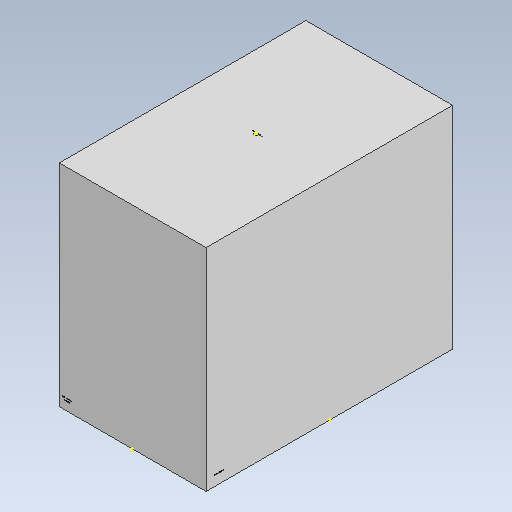
# Autodesk Inventor part: wheelchair_extended_box
Saved by Autodesk Inventor 2021 (Build 250183000, 183)
## iProperties
Created: 2021-05-27
Part Number: wheelchair_extended_box
Material: Generic
Document SubType Name: Modeling
Designer: Watchdog
Density: 1 g/cm^3
Appearance: Default
Author: Watchdog
Autodesk Inventor part; units mm, degrees
ref_plane "YZ Plane" through (0, 0, 0) normal (1, 0, 0) x (0, 1, 0)
ref_plane "XZ Plane" through (0, 0, 0) normal (0, 1, 0) x (-1, 0, 0)
ref_plane "XY Plane" through (0, 0, 0) normal (0, 0, 1) x (1, 0, 0)
sketch "Sketch1" plane through (0, 0, 0) normal (0, 1, 0) x (-1, 0, 0)
  line L0 (317.5, -533.5) -> (-317.5, -533.5)
  line L1 (-317.5, -533.5) -> (-317.5, 533.5)
  line L2 (-317.5, 533.5) -> (317.5, 533.5)
  line L3 (317.5, 533.5) -> (317.5, -533.5)
  point P0 (0, 0)
  dimension "d0" = 635
  dimension "d1" = 1067
  dimension "d2" = 533.5
  dimension "d3" = 317.5
  constraints: 8 end point, 2 parallel, 1 horizontal, 1 perpendicular
  measures "d0" distance of L0.start L0.end
  measures "d1" distance of L0.end L1.end
  measures "d2" distance from line of point (0, 0) L0
  measures "d3" distance from line of point (0, 0) L3
extrude "Extrusion1" add sketch "Sketch1" along normal blind 914
sketch "Sketch2" plane through (-317.5, 0, 533.5) normal (0, 0, 1) x (1, 0, 0)
  line L0 (18.3428, 49.3539) -> (47.3747, 49.3539) construction
  line L1 (47.3747, 49.3539) -> (47.3747, 42.9969) construction
  line L2 (47.3747, 42.9969) -> (18.3428, 42.9969) construction
  line L3 (18.3428, 42.9969) -> (18.3428, 49.3539) construction
  point P0 (317.5, 0)
  constraints: 2 other
sketch "Sketch3" plane through (-317.5, 0, -533.5) normal (-1, 0, 0) x (0, 0, 1)
  line L0 (30.8104, 48.5767) -> (82.087, 48.5767) construction
  line L1 (82.087, 48.5767) -> (82.087, 42.2296) construction
  line L2 (82.087, 42.2296) -> (30.8104, 42.2296) construction
  line L3 (30.8104, 42.2296) -> (30.8104, 48.5767) construction
  point P0 (533.5, 0)
  constraints: 2 other
sketch "Sketch4" plane through (317.5, 0, 533.5) normal (1, 0, 0) x (0, 0, -1)
  line L0 (32.5592, 45.8564) -> (78.0917, 45.8564) construction
  line L1 (78.0917, 45.8564) -> (78.0917, 29.6042) construction
  line L2 (78.0917, 29.6042) -> (32.5592, 29.6042) construction
  line L3 (32.5592, 29.6042) -> (32.5592, 45.8564) construction
  point P0 (533.5, 0)
  constraints: 2 other
sketch "Sketch5" plane through (317.5, 0, -533.5) normal (0, 0, -1) x (-1, 0, 0)
  line L0 (6.4578, 53.0458) -> (51.9903, 53.0458) construction
  line L1 (51.9903, 53.0458) -> (51.9903, 36.7836) construction
  line L2 (51.9903, 36.7836) -> (6.4578, 36.7836) construction
  line L3 (6.4578, 36.7836) -> (6.4578, 53.0458) construction
  point P0 (317.5, 0)
  constraints: 2 other
sketch "Sketch6" plane through (0, 914, 0) normal (0, 1, 0) x (1, 0, 0)
  line L0 (-31.9661, 8.1609) -> (33.1319, 8.1609) construction
  line L1 (33.1319, 8.1609) -> (33.1319, 1.8038) construction
  line L2 (33.1319, 1.8038) -> (-31.9661, 1.8038) construction
  line L3 (-31.9661, 1.8038) -> (-31.9661, 8.1609) construction
  point P0 (0, 0)
  constraints: 2 other
sketch "Sketch7" plane through (0, 0, 0) normal (0, -1, 0) x (1, 0, 0)
  line L0 (-23.7378, 6.995) -> (21.7947, 6.995) construction
  line L1 (21.7947, 6.995) -> (21.7947, -9.277) construction
  line L2 (21.7947, -9.277) -> (-23.7378, -9.277) construction
  line L3 (-23.7378, -9.277) -> (-23.7378, 6.995) construction
  point P0 (0, 0)
  dimension "d4" = 914
  constraints: 2 other
equation "\"d0\" = y"
equation "\"d1\" = x"
equation "\"d2\" = 0.5 * d1"
equation "\"d3\" = 0.5 * d0"
equation "\"d4\" = z"
equation "\"x\" = wheelchair_deployed_length"
equation "\"y\" = wheelchair_deployed_width"
equation "\"z\" = wheelchair_deployed_height"
equation "\"hoop_angle_z\" = 45deg"
equation "\"hoop_bearing_length\" = 5deg"
equation "\"hoop_cable_diam\" = 5"
equation "\"hoop_cable_pulley_diam\" = 22"
equation "\"hoop_thickness_large\" = 4"
equation "\"hoop_thickness_medium\" = 3.2"
equation "\"hoop_thickness_small\" = 2"
equation "\"hoop_width_large\" = 51"
equation "\"hoop_width_medium\" = 33.7"
equation "\"hoop_width_small\" = 25.4"
equation "\"rack_tooth_addendum\" = 5"
equation "\"rack_tooth_dedendum\" = 5"
equation "\"rack_tooth_thickness\" = 5"
equation "\"secure_arm_angle\" = 35deg"
equation "\"secure_arm_radii\" = 9"
equation "\"support_baseClamp_platformLengthBuffer\" = 35"
equation "\"support_baseClamp_platformThickness\" = 15"
equation "\"support_baseClamp_platformWidthBuffer\" = 0"
equation "\"support_baseClamp_sleeveHoleDiameter\" = 12"
equation "\"support_baseClamp_sleeveSweepTerminationAngle\" = 55deg"
equation "\"support_baseClamp_thickness\" = 8"
equation "\"support_frame_endHoleBuffer\" = 25"
equation "\"support_frame_squareBarFillet\" = 2"
equation "\"support_frame_squareBarThickness\" = 5"
equation "\"hoop_tabs_thickness\" = 6"
equation "\"hoop_tabs_hole\" = 12"
equation "\"wheelchair_deployed_width\" = 635"
equation "\"wheelchair_deployed_length\" = 1067"
equation "\"wheelchair_deployed_height\" = 914"
equation "\"sm_varx_member_tolerance\" = 0.5"
equation "\"sm_varx_pinPlate_holeDiameter\" = 5"
equation "\"sm_varx_pinPlate_thickness\" = 5"
equation "\"sm_varx_squareBarThickness\" = 2.5"
equation "\"hoop_bushing23_radialInterference\" = 0"
equation "\"hoop_bushing12_radialInterference\" = 0"
equation "\"hoop_bushing12_od\" = -2 * hoop_thickness_large + hoop_width_large + hoop_bushing12_radialInterference"
equation "\"hoop_bushing23_od\" = -2 * hoop_thickness_medium + hoop_width_medium + hoop_bushing23_radialInterference"
body "Solid1"
